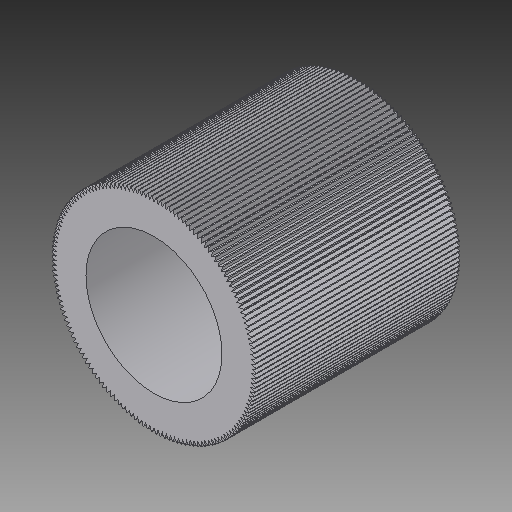
# Autodesk Inventor part: Roue dente
Saved by Autodesk Inventor 2017 (Build 210142000, 142)
## iProperties
Company: FABLAB Frenchmakers
Part Number: Roue dente
Material: ----------
Document SubType Name: Modeling
Designer: FABLAB Frenchmakers
Density: 7.86 g/cm^3
Appearance: Métal - Acier
Mass: 5.5609 g
Surface Area: 14.7111 cm^2
Volume: 0.707494 cm^3
Project: 1420 Vauban 3D XL
Catalog Web Link: http://frenchmakers.com/
Stock Number: 1420-05-13
Autodesk Inventor part; units mm, degrees
ref_plane "YZ Plane" through (0, 0, 0) normal (1, 0, 0) x (0, 1, 0)
ref_plane "XZ Plane" through (0, 0, 0) normal (0, 1, 0) x (-1, 0, 0)
ref_plane "XY Plane" through (0, 0, 0) normal (0, 0, 1) x (1, 0, 0)
sketch "Esquisse1" plane through (0, 0, 0) normal (0, 0, 1) x (1, 0, 0)
  circle A0 centre (0, 0) radius 4
  circle A1 centre (0, 0) radius 6
  dimension "d0" = 8
  dimension "d1" = 12
  constraints: 2 centre point, 2 coincident
  measures "d0" diameter of A0
  measures "d1" diameter of A1
extrude "Extrusion1" add sketch "Esquisse1" along normal mid plane 12
sketch "Esquisse2" plane through (0, 0, 6) normal (0, 0, 1) x (1, 0, 0)
  line L0 (-0.8284, 7.75) -> (0, 5.75)
  line L1 (0, 5.75) -> (0.8284, 7.75)
  line L2 (0.8284, 7.75) -> (-0.8284, 7.75)
  point P0 (0, 0)
  dimension "d4" = 5.75
  dimension "d5" = 45
  dimension "d6" = 2
  constraints: 6 end point, 1 equal length, 1 horizontal, 1 vertical alignment
  measures "d4" distance of point (0, 0) L0.end
  measures "d5" angle of L0 L1
  measures "d6" distance from line of L0.end L2
extrude "Extrusion2" cut sketch "Esquisse2" against normal through all
pattern_circular "Réseau circulaire1" count 150 over 360 about axis through (0, 0, 0) along (0, 0, 1) of "Extrusion2"
